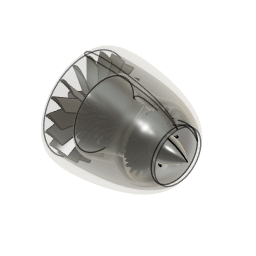
Pearl 700 High Bypass Turbofan Engine_ (Autodesk Fusion 360 design; units mm, degrees)
Autodesk Fusion 360 part; units mm, degrees
sketch "Sketch1" plane through (0, 0, 0) normal (0, 1, 0) x (1, 0, 0)
  line L0 (-500, 0) -> (400, 0)
  line L1 (-380, -70) -> (-249.2821, -88.2176)
  spline S0 degree 5 poles (-380, -70) (-387.6525, -66.787) (-402.6258, -60.4089) (-424.0913, -50.9858) (-450.585, -38.7296) (-478.4226, -24.1739) (-493.8079, -13.5263) (-499.5289, -6.383) (-500.3433, -2.0552) (-500, 0) knots 0 0 0 0 0 0 0.2 0.4 0.6 0.8 1 1 1 1 1 1
  line L2 (-500.4638, -2.7764) -> (-499.5362, 2.7764)
  line L3 (-249.2821, -88.2176) -> (-249.2821, -61.9175)
  line L4 (-130.4277, -47.1311) -> (-30.4277, -47.1311)
  line L5 (-30.4277, -47.1311) -> (-30.4277, -32.1311)
  line L6 (-30.4277, -32.1311) -> (59.5723, -32.1311)
  line L7 (59.5723, -32.1311) -> (59.5723, -47.1311)
  line L8 (59.5723, -47.1311) -> (159.5723, -47.1311)
  spline S1 degree 5 poles (159.5723, -47.1311) (164.4894, -56.919) (176.3157, -73.0113) (200.0252, -86.7081) (241.4203, -87.0313) (300.401, -67.9808) (345.8196, -43.851) (375.232, -22.8891) (392.1867, -7.8133) (400, 0) knots 0 0 0 0 0 0 0.2 0.4 0.6 0.8 1 1 1 1 1 1
  line L9 (149.5723, -27.2251) -> (169.5723, -67.037)
  line L10 (380, -20) -> (420, 20)
  spline S2 degree 5 poles (-249.2821, -61.9175) (-244.2555, -61.8853) (-234.0051, -61.642) (-218.039, -60.7409) (-195.9607, -58.6278) (-169.0985, -55.0664) (-150.3411, -51.9003) (-139.0818, -49.5067) (-133.0641, -47.9212) (-130.4277, -47.1311) knots 0 0 0 0 0 0 0.2 0.4 0.6 0.8 1 1 1 1 1 1
  line L11 (-267.5979, -62.0348) -> (-230.9663, -61.8002)
  line L12 (-140, -50) -> (-120.8554, -44.2621)
  dimension "d1" = 900
  dimension "d2" = 500
  dimension "d4" = 100
  dimension "d5" = 15
  dimension "d6" = 15
  dimension "d7" = 90
  dimension "d8" = 100
  constraint horizontal L0
  constraint midpoint L0.start L2
  constraint vertical L3
  constraint parallel L0 L4
  constraint perpendicular L0 L5
  constraint perpendicular L5 L6
  constraint perpendicular L0 L7
  constraint perpendicular L7 L8
  constraint midpoint L8.end L9
  constraint midpoint L0.end L10
  constraint midpoint L3.end L11
  constraint midpoint L4.start L12
  measures "d1" distance of L0.start L0.end
  measures "d2" distance of origin L0.start
  measures "d4" distance of L4.start L4.end
  measures "d5" distance of L4.end L5.end
  measures "d6" distance of L6.end L7.end
  measures "d7" distance of L5.end L6.end
  measures "d8" distance of L7.end L8.end
revolve "Revolve1" add sketch "Sketch1" angle 360 about axis through (-500, 0, 0) along (1, 0, 0) makes body 1
ref_plane "WorkPlane1" through (0, 0, 300) normal (0, 0, 1) x (1, 0, 0)
sketch "Sketch2" plane through (0, 0, 300) normal (0, 0, 1) x (1, 0, 0)
  spline S0 degree 5 poles (-372.0669, 20.1106) (-370.5749, 21.8475) (-366.6645, 24.3623) (-358.0223, 25.2599) (-341.7121, 21.5007) (-316.0135, 11.3034) (-292.8481, 0.4472) (-274.4896, -8.7142) (-261.8415, -15.2453) (-255.4151, -18.6168) knots 0 0 0 0 0 0 0.2 0.4 0.6 0.8 1 1 1 1 1 1
  line L0 (-375.1379, 16.5354) -> (-368.9958, 23.6858)
  spline S1 degree 5 poles (-372.0669, 20.1106) (-373.9909, 17.8708) (-376.832, 14.2112) (-378.0745, 11.1794) (-373.7712, 10.8646) (-356.4386, 11.0015) (-328.8504, 6.069) (-297.0898, -3.5078) (-270.2516, -13.0531) (-255.4151, -18.6168) knots 0 0 0 0 0 0 0.2 0.4 0.6 0.8 1 1 1 1 1 1
  line L1 (-368.9958, 23.6858) -> (-375.1379, 16.5354)
  line L2 (-295.4151, -3.6168) -> (-215.4151, -33.6168)
  constraint midpoint S0.start L0
  constraint midpoint S0.start L1
  constraint midpoint S0.end L2
  constraint coincident L0.start L1.end
extrude "Extrude1" add sketch "Sketch2" against normal blind 250 bodies 1
pattern_circular "C-Pattern1" count 18 over 360 about axis through (1.75, 0, 0) along (1, 0, 0) of "Extrude1"
ref_plane "WorkPlane2" through (0, 0, 200) normal (0, 0, 1) x (1, 0, 0)
sketch "Sketch3" plane through (0, 0, 200) normal (0, 0, 1) x (1, 0, 0)
  spline S0 degree 5 poles (-222.5778, -2.3707) (-221.665, -2.1864) (-220.3562, -1.7973) (-219.9413, -1.1516) (-222.0577, -0.1841) (-227.6649, 1.1437) (-233.6042, 2.2641) (-238.6077, 3.1263) (-242.1715, 3.7102) (-244.0104, 4.0044) knots 0 0 0 0 0 0 0.2 0.4 0.6 0.8 1 1 1 1 1 1
  line L0 (-223.65, -2.5871) -> (-221.5056, -2.1542)
  spline S1 degree 5 poles (-222.5778, -2.3707) (-222.4343, -2.3417) (-222.4393, -2.2178) (-223.3224, -1.8342) (-226.0093, -0.9818) (-231.0426, 0.4618) (-235.8911, 1.8024) (-239.8379, 2.8779) (-242.5981, 3.6241) (-244.0104, 4.0044) knots 0 0 0 0 0 0 0.2 0.4 0.6 0.8 1 1 1 1 1 1
  line L1 (-222.7464, -2.4047) -> (-222.4092, -2.3367)
  constraint midpoint S0.start L0
  constraint midpoint S0.start L1
  constraint coincident L0 L1.end
extrude "Extrude3" add sketch "Sketch3" against normal blind 140 bodies 1
pattern_circular "C-Pattern2" count 20 over 360 about axis through (1.75, 0, 0) along (1, 0, 0) of "Extrude3"
ref_plane "WorkPlane3" through (0, 0, 175) normal (0, 0, 1) x (1, 0, 0)
sketch "Sketch5" plane through (0, 0, 175) normal (0, 0, 1) x (1, 0, 0)
  spline S0 degree 5 poles (-210, -1.9258) (-210, -2.7292) (-209.661, -4.0023) (-208.1362, -4.9115) (-204.3516, -4.4238) (-197.6804, -2.1037) (-191.3952, 0.3337) (-186.3262, 2.188) (-182.7999, 3.4) (-181, 4) knots 0 0 0 0 0 0 0.2 0.4 0.6 0.8 1 1 1 1 1 1
  line L0 (-210, -1.0859) -> (-210, -2.7657)
  spline S1 degree 5 poles (-210, -1.9258) (-210, -1.3325) (-209.5638, -0.2068) (-207.602, 1.2999) (-202.8127, 2.9593) (-194.9839, 4.3937) (-188.654, 4.8565) (-184.5087, 4.6673) (-182.1089, 4.268) (-181, 4) knots 0 0 0 0 0 0 0.2 0.4 0.6 0.8 1 1 1 1 1 1
  line L1 (-183.0984, 4.5071) -> (-178.9016, 3.4929)
  line L2 (-210, -2.7657) -> (-210, -1.0859)
  line L3 (-184, 3) -> (-178, 5)
  constraint midpoint S0.start L0
  constraint midpoint S0.end L1
  constraint midpoint S0.start L2
  constraint coincident L0.start L2.end
  constraint midpoint S0.end L3
extrude "Extrude4" add sketch "Sketch5" against normal blind 140 bodies 1
pattern_circular "C-Pattern3" count 20 over 360 about axis through (1.75, 0, 0) along (1, 0, 0) of "Extrude4"
ref_plane "WorkPlane4" through (0, 0, 150) normal (0, 0, 1) x (1, 0, 0)
sketch "Sketch6" plane through (0, 0, 150) normal (0, 0, 1) x (1, 0, 0)
  spline S0 degree 5 poles (-145, -5) (-148.1383, -3.8231) (-153.8669, -1.758) (-160.8167, 0.4748) (-167.2361, 2.0116) (-171.9993, 2.6952) (-174.0586, 3.1651) (-174.8288, 3.8857) (-175, 4.5911) (-175, 5) knots 0 0 0 0 0 0 0.2 0.4 0.6 0.8 1 1 1 1 1 1
  spline S1 degree 5 poles (-175, 5) (-175, 5.5053) (-174.6498, 6.2517) (-173.0747, 6.5794) (-169.1647, 5.6509) (-162.2693, 2.9754) (-155.7676, 0.0915) (-150.5192, -2.3521) (-146.8655, -4.0979) (-145, -5) knots 0 0 0 0 0 0 0.2 0.4 0.6 0.8 1 1 1 1 1 1
  line L0 (-175, 4.2229) -> (-175, 5.7771)
  line L1 (-137, -8) -> (-153, -2)
  line L2 (-175, 4.2229) -> (-175, 5.7771)
  constraint midpoint S0.end L0
  constraint midpoint S0.start L1
  constraint midpoint S0.end L2
  constraint parallel L0 L2
extrude "Extrude5" add sketch "Sketch6" against normal blind 100 bodies 1
pattern_circular "C-Pattern4" count 20 over 360 about axis through (1.75, 0, 0) along (1, 0, 0) of "Extrude5"
ref_plane "WorkPlane5" through (0, 0, 125) normal (0, 0, 1) x (1, 0, 0)
sketch "Sketch7" plane through (0, 0, 150) normal (0, 0, 1) x (1, 0, 0)
  spline S0 degree 5 poles (-120.4333, -0.3331) (-120.1251, -0.1359) (-119.5158, 0.2225) (-118.6224, 0.6524) (-117.3448, 1.0475) (-114.7863, 1.3973) (-110.9949, 1.6854) (-106.5389, 1.9638) (-102.7256, 2.1859) (-100.6082, 2.3061) knots 0 0 0 0 0 0 0.2 0.4 0.6 0.8 1 1 1 1 1 1
  spline S1 degree 5 poles (-40.2532, 1.8602) (-41.7226, 1.5229) (-44.5783, 0.9592) (-48.6129, 0.4467) (-53.465, 0.2813) (-58.2518, 0.2537) (-60.4341, -0.2622) (-60.6847, -1.2716) (-60.1376, -2.2821) (-59.6853, -2.8717) knots 0 0 0 0 0 0 0.2 0.4 0.6 0.8 1 1 1 1 1 1
  spline S2 degree 5 poles (-69.5706, -1.3613) (-71.0328, -0.8428) (-73.8795, 0.1452) (-77.9166, 1.4803) (-82.8013, 2.9463) (-87.6705, 3.999) (-89.9533, 3.8243) (-90.3027, 2.834) (-89.8331, 1.7307) (-89.4225, 1.0683) knots 0 0 0 0 0 0 0.2 0.4 0.6 0.8 1 1 1 1 1 1
  spline S3 degree 5 poles (-120.4333, -0.3331) (-121.0081, -0.7009) (-121.79, -1.3777) (-121.8603, -2.2163) (-120.0274, -2.965) (-115.4157, -3.0285) (-110.3184, -1.9714) (-105.7619, -0.2507) (-102.383, 1.3741) (-100.6082, 2.3061) knots 0 0 0 0 0 0 0.2 0.4 0.6 0.8 1 1 1 1 1 1
  spline S4 degree 5 poles (-89.4225, 1.0683) (-89.1537, 0.6346) (-88.4628, -0.1346) (-86.9669, -0.994) (-84.1802, -1.6323) (-79.8179, -1.8671) (-75.8967, -1.7786) (-72.7929, -1.6079) (-70.656, -1.4507) (-69.5706, -1.3613) knots 0 0 0 0 0 0 0.2 0.4 0.6 0.8 1 1 1 1 1 1
  spline S5 degree 5 poles (-59.6853, -2.8717) (-59.3403, -3.3216) (-58.5241, -4.0347) (-56.9217, -4.5453) (-54.1332, -4.2622) (-49.9242, -2.839) (-46.202, -1.1756) (-43.2764, 0.2702) (-41.2702, 1.3165) (-40.2532, 1.8602) knots 0 0 0 0 0 0 0.2 0.4 0.6 0.8 1 1 1 1 1 1
  line L0 (-119.6827, 0.1472) -> (-121.1838, -0.8133)
  line L1 (-121.1838, -0.8133) -> (-119.6827, 0.1472)
  line L2 (-106, 2) -> (-95.2163, 2.6122)
  line L3 (-90, 2) -> (-88.845, 0.1365)
  line L4 (-90, 2) -> (-88.845, 0.1365)
  line L5 (-60.363, -1.9881) -> (-59.0076, -3.7553)
  line L6 (-60.363, -1.9881) -> (-59.0076, -3.7553)
  line L7 (-36.5064, 2.7204) -> (-44, 1)
  line L8 (-105, 0) -> (-96.2163, 4.6122)
  point P0 (-130.4277, 0)
  point P1 (-30.4277, 0)
  dimension "d33" = 20
  dimension "d34" = 20
  dimension "d35" = 20
  dimension "d36" = 10
  dimension "d37" = 10
  dimension "d38" = 10
  constraint midpoint S0.start L0
  constraint midpoint S0.start L1
  constraint coincident L0 L1.end
  constraint midpoint S0.end L2
  constraint midpoint S2.end L3
  constraint midpoint S2.end L4
  constraint coincident L3.end L4.end
  constraint midpoint S1.end L5
  constraint midpoint S1.end L6
  constraint coincident L5.end L6.end
  constraint midpoint S1.start L7
  constraint midpoint S0.end L8
  measures "d33" distance of S0.start S0.end
  measures "d34" distance of S2.start S2.end
  measures "d35" distance of S1.start S1.end
  measures "d36" distance of S0.start P0
  measures "d37" distance of S1.start P1
  measures "d38" distance of S1.end S2.start
extrude "Extrude6" add sketch "Sketch7" against normal blind 110 bodies 1
pattern_circular "C-Pattern5" count 20 over 360 about axis through (1.75, 0, 0) along (1, 0, 0) of "Extrude6"
sketch "Sketch8" plane through (0, 0, 125) normal (0, 0, 1) x (1, 0, 0)
  spline S0 degree 5 poles (65, -1.3844) (64.6734, -0.7623) (64.3956, 0.2801) (65.1037, 1.2387) (67.9585, 1.5041) (73.4438, 0.9244) (78.4742, 0.3255) (82.2657, 0.0592) (84.7607, 0) (86, 0) knots 0 0 0 0 0 0 0.2 0.4 0.6 0.8 1 1 1 1 1 1
  spline S1 degree 5 poles (65, -1.3844) (65.2108, -1.521) (65.8161, -1.7381) (67.2744, -1.8959) (70.1677, -1.8168) (74.8372, -1.3967) (79.0894, -0.9029) (82.4737, -0.4731) (84.8111, -0.1618) (86, 0) knots 0 0 0 0 0 0 0.2 0.4 0.6 0.8 1 1 1 1 1 1
  line L0 (65.4648, -2.2697) -> (64.5352, -0.4991)
  line L1 (64.5352, -1.0833) -> (65.4648, -1.6855)
  line L2 (83, 0) -> (89, 0)
  constraint midpoint S0.start L0
  constraint midpoint S0.start L1
  constraint midpoint S0.end L2
extrude "Extrude7" add sketch "Sketch8" against normal blind 80 bodies 1
extrude "Extrude9" add sketch "Sketch6" along normal blind 10 bodies 1
pattern_circular "C-Pattern6" count 20 over 360 about axis through (1.75, 0, 0) along (1, 0, 0) of "Extrude9"
pattern_circular "C-Pattern7" count 20 over 360 about axis through (1.75, 0, 0) along (1, 0, 0) of "Extrude7"
extrude "Extrude10" add 1 faces at (71.0187, -0.6548, 125) along direction (0, 0, 1) blind 25 on bodies 1 bodies 1
pattern_circular "C-Pattern8" count 20 over 360 about axis through (1.75, 0, 0) along (1, 0, 0) of "Extrude10"
sketch "Sketch9" plane through (0, 0, 0) normal (0, 0, 1) x (1, 0, 0)
  spline S0 degree 5 poles (100, 0) (99.2735, 0.7303) (98.1748, 1.9208) (97.5891, 2.897) (98.6666, 2.8498) (102.2661, 1.6264) (106.5321, 0.5646) (110.4658, 0.1027) (113.4314, 0) (115, 0) knots 0 0 0 0 0 0 0.2 0.4 0.6 0.8 1 1 1 1 1 1
  spline S1 degree 5 poles (100, 0) (100.227, -0.2282) (100.7337, -0.6568) (101.6516, -1.2163) (103.1936, -1.7863) (105.8021, -2.0778) (108.7052, -1.772) (111.552, -1.09) (113.7933, -0.4022) (115, 0) knots 0 0 0 0 0 0 0.2 0.4 0.6 0.8 1 1 1 1 1 1
  line L0 (101, -1.0052) -> (99, 1.0052)
  line L1 (99.4954, 0.5072) -> (100.5046, -0.5072)
  line L2 (112, -1) -> (118, 1)
  line L3 (111, 0) -> (119, 0)
  constraint midpoint S0.start L0
  constraint midpoint S0.start L1
  constraint midpoint S0.end L2
  constraint midpoint S0.end L3
extrude "Extrude11" add sketch "Sketch9" along normal blind 175 bodies 1
pattern_circular "C-Pattern9" count 20 over 360 about axis through (1.75, 0, 0) along (1, 0, 0) of "Extrude11"
sketch "Sketch10" plane through (0, 0, 200) normal (0, 0, 1) x (1, 0, 0)
  spline S0 degree 5 poles (125, 0) (125.177, 0.177) (125.5513, 0.4656) (126.1734, 0.7023) (127.1924, 0.6908) (129.2783, 0.3943) (132.2306, 0.1369) (135.5929, 0.0249) (138.4314, 0) (140, 0) knots 0 0 0 0 0 0 0.2 0.4 0.6 0.8 1 1 1 1 1 1
  spline S1 degree 5 poles (125, 0) (124.2731, -0.7269) (123.2066, -1.9685) (122.7676, -3.1951) (124.1835, -3.7342) (128.1735, -3.1918) (132.4551, -2.161) (136.0779, -1.1625) (138.6641, -0.4031) (140, 0) knots 0 0 0 0 0 0 0.2 0.4 0.6 0.8 1 1 1 1 1 1
  line L0 (126, 1) -> (124, -1)
  line L1 (124.6062, -0.3938) -> (125.3938, 0.3938)
  line L2 (136, 0) -> (144, 0)
  constraint midpoint S0.start L0
  constraint midpoint S0.start L1
  constraint midpoint S0.end L2
extrude "Extrude12" add sketch "Sketch10" against normal blind 200 bodies 1
pattern_circular "C-Pattern10" count 20 over 360 about axis through (1.75, 0, 0) along (1, 0, 0) of "Extrude12"
sketch "Sketch11" plane through (0, 0, 0) normal (0, 0, 1) x (1, 0, 0)
  spline S0 degree 5 poles (-232.867, 225.0947) (-231.8782, 224.4386) (-229.1624, 222.8657) (-222.8739, 219.7239) (-210.0404, 213.9627) (-186.7066, 204.2655) (-156.6159, 192.4976) (-121.0328, 179.5955) (-82.0975, 167.0921) (-42.3681, 156.7638) (-4.4677, 150.3509) (29.2955, 149.255) (57.3234, 154.2201) (79.0789, 165.0502) (95.612, 180.1722) (109.1676, 197.0086) (122.4812, 212.6275) (138.2356, 224.2478) (158.3466, 229.9098) (183.9678, 228.4498) (215.7253, 219.2538) (246.2349, 205.5308) (272.0007, 191.6537) (290.4542, 180.8157) (300, 175) knots 0 0 0 0 0 0 0.05 0.1 0.15 0.2 0.25 0.3 0.35 0.4 0.45 0.5 0.55 0.6 0.65 0.7 0.75 0.8 0.85 0.9 0.95 1 1 1 1 1 1
  spline S1 degree 5 poles (-232.867, 225.0947) (-232.637, 228.4383) (-231.4278, 234.5601) (-227.3664, 242.0466) (-217.4392, 248.6239) (-197.6675, 251.3428) (-171.2319, 249.2542) (-139.6031, 243.7865) (-104.6816, 236.7462) (-68.5402, 230.0457) (-33.1436, 225.4041) (-0.0764, 224.0565) (29.7326, 226.4558) (56.3088, 231.9488) (80.3609, 239.1158) (103.0046, 246.1186) (125.5009, 251.032) (148.9901, 252.1832) (174.2368, 248.4809) (201.7145, 239.2772) (231.675, 224.2542) (257.7095, 207.5005) (278.4027, 192.279) (292.7148, 180.9556) (300, 175) knots 0 0 0 0 0 0 0.05 0.1 0.15 0.2 0.25 0.3 0.35 0.4 0.45 0.5 0.55 0.6 0.65 0.7 0.75 0.8 0.85 0.9 0.95 1 1 1 1 1 1
  point P0 (-162.867, 195.0947)
  point P1 (61.909, 157.8434)
  point P2 (127.133, 215.0947)
  point P3 (-200, 250)
  point P4 (0, 225)
  point P5 (125, 250)
revolve "Revolve2" add sketch "Sketch11" angle 360 about axis through (1.75, 0, 0) along (1, 0, 0) separate body makes body 2
sketch "Sketch12" plane through (0, 0, 0) normal (0, 1, 0) x (1, 0, 0)
  spline S0 degree 5 poles (-374.576, -312.7671) (-354.2303, -313.2891) (-314.0414, -314.0739) (-255.2652, -314.4737) (-179.9616, -313.4262) (-91.3339, -309.2791) (-8.8391, -301.9688) (66.7416, -291.0923) (134.6439, -276.2556) (194.3497, -257.1912) (245.9911, -233.9674) (281.1953, -212.2376) (304.3429, -194.2611) (318.3515, -181.5427) (325, -175) knots 0 0 0 0 0 0 0.1 0.2 0.3 0.4 0.5 0.6 0.7 0.8 0.9 1 1 1 1 1 1
  spline S1 degree 5 poles (-374.576, -312.7671) (-376.1691, -317.1347) (-377.7095, -325.3898) (-375.0813, -336.3322) (-361.6368, -348.0219) (-328.464, -357.7464) (-280.4834, -362.6709) (-220.4694, -363.0087) (-151.9063, -359.0343) (-78.6623, -351.0522) (-4.6438, -339.3685) (66.5337, -324.2765) (131.8404, -306.048) (189.2653, -284.9378) (237.7726, -261.1745) (276.9392, -234.9434) (300.7754, -212.0913) (314.4933, -193.9375) (321.8036, -181.3871) (325, -175) knots 0 0 0 0 0 0 0.066667 0.133333 0.2 0.266667 0.333333 0.4 0.466667 0.533333 0.6 0.666667 0.733333 0.8 0.866667 0.933333 1 1 1 1 1 1
  point P0 (138.4706, -273.6137)
  point P1 (-350, -350)
  point P2 (92.6342, -316.3622)
revolve "Revolve3" add sketch "Sketch12" angle 360 about axis through (1.75, 0, 0) along (1, 0, 0) separate body makes body 3
extrude "Extrude8" [suppressed]
ref_plane "WorkPlane6" through (0, 0, 160) normal (0, 0, 1) x (1, 0, 0)
extrude "Extrude2" [suppressed]
